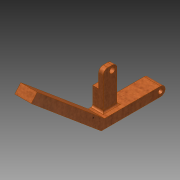
# Autodesk Inventor part: Swinging_connection
Saved by Autodesk Inventor 2015 (Build 190159000, 159)
## iProperties
Created: 2017-02-21
Part Number: Swinging_connection
Material: Wood (Cherry)
Document SubType Name: Modeling
Designer: Guy
Density: 0.63 g/cm^3
Appearance: Cherry - Natural Low Gloss
Mass: 13.2068 g
Surface Area: 69.6944 cm^2
Volume: 20.9632 cm^3
Author: Guy
Autodesk Inventor part; units mm, degrees
ref_plane "YZ Plane" through (0, 0, 0) normal (1, 0, 0) x (0, 1, 0)
ref_plane "XZ Plane" through (0, 0, 0) normal (0, 1, 0) x (-1, 0, 0)
ref_plane "XY Plane" through (0, 0, 0) normal (0, 0, 1) x (1, 0, 0)
sketch "Sketch1" plane through (0, 0, 0) normal (0, 0, 1) x (1, 0, 0)
  line L0 (0, 0) -> (-65.3369, 0)
  line L1 (0, 0) -> (0, -10)
  line L2 (0, -10) -> (-70, -10)
  circle A0 centre (-5, -5) radius 2.5
  line L3 (-65.3369, 0) -> (-126.6183, 73.0323)
  line L4 (-126.6183, 73.0323) -> (-134.2788, 66.6044)
  line L5 (-134.2788, 66.6044) -> (-70, -10)
  line L6 (-5, -5) -> (86.9903, 72.1891)
  line L7 (-5, -5) -> (-134.7228, 149.5976)
  dimension "d1" = 5
  dimension "d2" = 10
  dimension "d3" = 5
  dimension "d4" = 5
  dimension "d50" = 70
  dimension "d51" = 130
  dimension "d52" = 10
  dimension "d53" = 100
  dimension "d55" = 40
  constraints: 16 end point, 2 horizontal, 2 perpendicular, 1 centre point, 1 parallel, 1 vertical
  measures "d1" diameter of A0
  measures "d2" distance between parallel lines of L2 L0
  measures "d3" distance from line of L6.start L0
  measures "d4" distance from line of L6.start L1
  measures "d50" distance from line of L2.end L1
  measures "d51" angle of L0 L3
  measures "d52" distance of L3.end L4.end
  measures "d53" distance from line of L2.end L4
  measures "d55" angle of L2 L6
extrude "Extrusion1" add sketch "Sketch1" along normal blind 18 contours L1 L6 A0 L7 L0 | L7 A0 L6 L1 L2 L5 L4 L3 L0
fillet "Fillet5" radius 5 2 edges at (0, 0, 9) (0, -10, 9)
sketch "Sketch5" plane through (-70, 0, 0) normal (0, 1, 0) x (1, 0, 0)
  line L0 (9.6631, 0) -> (24.6631, 0)
  line L1 (24.6631, 0) -> (24.6631, -11.5)
  line L2 (24.6631, -11.5) -> (9.6631, -11.5)
  line L3 (9.6631, -11.5) -> (9.6631, 0)
  line L4 (65, -18) -> (4.6631, -18) projected
  line L5 (0, 0) -> (0, -18) projected
  line L6 (65, 0) -> (4.6631, 0) projected
  line L7 (4.6631, 0) -> (4.6631, -18) projected
  point P0 (70, 0)
  point P1 (0, -3.5)
  dimension "d31" = 15
  dimension "d33" = 6.5
  dimension "d54" = 20
  constraints: 8 end point, 2 parallel, 1 horizontal, 1 perpendicular, 1 point on line
  measures "d31" distance between parallel lines of L3 L1
  measures "d33" distance between parallel lines of L4 L2
  measures "d54" distance between parallel lines of L7 L1
extrude "Extrusion5" add sketch "Sketch5" along normal blind 30
sketch "Sketch6" plane through (-45.3369, 0, 11.5) normal (0, 0, 1) x (1, 0, 0)
  circle A0 centre (-5, 25) radius 3
  line L0 (-15, 30) -> (0, 30) projected
  line L1 (0, 0) -> (0, 30) projected
  point P0 (45.3369, 0)
  dimension "d37" = 6
  dimension "d38" = 5
  dimension "d39" = 5
  constraints: 1 centre point
  measures "d37" diameter of A0
  measures "d38" distance from line of A0.centre L0
  measures "d39" distance from line of A0.centre L1
extrude "Extrusion6" cut sketch "Sketch6" against normal up to next
sketch "Sketch7" plane through (-60.3369, 0, 0) normal (-1, 0, 0) x (0, 0, 1)
  line L0 (0, 30) -> (6.5, 30)
  line L1 (0, 10) -> (0, 30)
  line L2 (6.5, 30) -> (6.5, 10)
  line L3 (6.5, 10) -> (0, 10)
  line L4 (0, 0) -> (0, 30) projected
  line L5 (11.5, 0) -> (11.5, 30) projected
  line L6 (0, 30) -> (11.5, 30) projected
  dimension "d42" = 5
  dimension "d44" = 20
  constraints: 8 end point, 2 parallel, 1 horizontal, 1 perpendicular, 1 vertical
  measures "d42" distance between parallel lines of L5 L2
  measures "d44" distance from line of L2.end L0
extrude "Extrusion7" cut sketch "Sketch7" against normal up to next
fillet "Fillet8" radius 5 2 edges at (-45.3369, 30, 9) (-60.3369, 30, 9)
fillet "Fillet9" radius 2 3 edges at (-60.3369, 0, 5.75) (-52.8369, 0, 11.5) (-45.3369, 0, 5.75)
sketch "Sketch8" plane through (-70, -10, 0) normal (-0.7660444, -0.6427876, 0) x (0, 0, 1)
  circle A0 centre (9, 90) radius 6
  line L0 (0, 100) -> (18, 100) projected
  line L1 (18, 100) -> (18, 0) projected
  point P0 (0, -37.3347)
  dimension "d56" = 12
  dimension "d57" = 10
  dimension "d58" = 9
  constraints: 1 centre point
  measures "d56" diameter of A0
  measures "d57" distance from line of L0 A0.centre
  measures "d58" distance from line of L1 A0.centre
extrude "Extrusion8" add sketch "Sketch8" along normal blind 10
fillet "Fillet11" radius 2 2 edges at (-135.5113, 52.5161, 3) (-127.8509, 58.944, 3)
body "Solid1"
